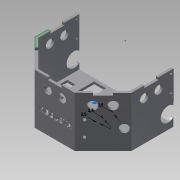
# Autodesk Inventor part: Kepala Depan 2
Saved by Autodesk Inventor 2015 SP1 (Build 190203100, 203)
## iProperties
Created: 2015-02-01
Part Number: Kepala Depan 2
Material: Generic
Document SubType Name: Modeling
Designer: Rafi Kurnia Putra
Density: 1 g/cm^3
Appearance: Default
Mass: 71.957 g
Surface Area: 473.113 cm^2
Volume: 71.957 cm^3
Author: Rafi Kurnia Putra
Autodesk Inventor part; units mm, degrees
ref_plane "YZ Plane" through (0, 0, 0) normal (1, 0, 0) x (0, 1, 0)
ref_plane "XZ Plane" through (0, 0, 0) normal (0, 1, 0) x (-1, 0, 0)
ref_plane "XY Plane" through (0, 0, 0) normal (0, 0, 1) x (1, 0, 0)
sketch "Sketch1" plane through (0, 0, 0) normal (0, 1, 0) x (-1, 0, 0)
  line L0 (60.406, -52.6639) -> (25.0211, -88.0488)
  line L1 (60.406, -52.6639) -> (60.406, 0)
  line L2 (-60.4057, -52.6639) -> (-60.4057, 0)
  line L3 (25.0211, -88.0488) -> (-25.0207, -88.0488)
  line L4 (-60.4057, 0) -> (60.406, 0)
  line L5 (-25.0207, -88.0488) -> (-60.4057, -52.6639)
  line L6 (57.406, 0) -> (57.406, -51.4212)
  line L7 (57.406, -51.4212) -> (23.7784, -85.0488)
  line L8 (23.7784, -85.0488) -> (-23.7781, -85.0488)
  line L9 (-23.7781, -85.0488) -> (-57.4057, -51.4212)
  line L10 (-57.4057, -51.4212) -> (-57.4057, 0)
  point P0 (0, -6165561.8884)
  point P1 (0, 0)
  point P2 (0.0002, 0)
  dimension "d195" = 120.8117
  dimension "d198" = 50.0418
  dimension "d199" = 50.0418
  dimension "d200" = 50.0418
  dimension "d201" = 52.6639
  dimension "d202" = 52.6639
  dimension "d204" = 3
  dimension "d205" = 51.4212
  dimension "d206" = 47.5566
  dimension "d207" = 47.5566
  dimension "d208" = 47.5566
  dimension "d209" = 51.4212
  dimension "d210" = 135
  dimension "d211" = 135
  dimension "d212" = 135
  dimension "d213" = 135
  dimension "d214" = 135
  dimension "d215" = 135
  dimension "d216" = 135
  dimension "d217" = 135
  dimension "d218" = 3
  dimension "d219" = 3
  dimension "d220" = 3
  constraints: 22 end point, 2 point on line, 1 horizontal, 1 horizontal alignment, 1 midpoint, 1 vertical, 3 other
  measures "d195" distance between parallel lines of L2 L1
  measures "d198" distance of L0.end L3.end
  measures "d199" distance of L0.start L0.end
  measures "d200" distance of L3.end L2.start
  measures "d201" distance of L0.start L1.end
  measures "d202" distance of L2.start L2.end
  measures "d204" distance between parallel lines of L6 L1
  measures "d205" distance of L6.start L6.end
  measures "d206" distance of L6.end L7.end
  measures "d207" distance of L7.end L8.end
  measures "d208" distance of L8.end L9.end
  measures "d209" distance of L9.end L10.end
  measures "d210" angle of L7 L6
  measures "d211" angle of L8 L7
  measures "d212" angle of L9 L8
  measures "d213" angle of L10 L9
  measures "d214" angle of L0 L1
  measures "d215" angle of L3 L0
  measures "d216" angle of L5 L3
  measures "d217" angle of L2 L5
  measures "d218" distance between parallel lines of L7 L0
  measures "d219" distance between parallel lines of L8 L3
  measures "d220" distance between parallel lines of L5 L9
extrude "Extrusion8" add sketch "Sketch1" along normal blind 3
extrude "Extrusion9" add sketch "Sketch1" against normal blind 60 contours L0 L3 L5 L2 L4 L10 L9 L8 L7 L6 L1
sketch "Sketch10" plane through (0, 3, 0) normal (0, 1, 0) x (1, 0, 0)
  circle A0 centre (13.2193, 32.61) radius 1.75
  circle A1 centre (39.7053, 32.61) radius 1.75
  circle A2 centre (39.7053, 8.2) radius 1.75
  circle A3 centre (13.2193, 8.2) radius 1.75
  circle A4 centre (20, 57.8773) radius 1.75
  circle A5 centre (-20, 57.8773) radius 1.75
  point P0 (0, 0)
  dimension "d115" = 3.5
  dimension "d116" = 3.5
  dimension "d117" = 3.5
  dimension "d118" = 3.5
  dimension "d119" = 3.5
  dimension "d120" = 3.5
  constraints: 6 centre point, 1 coincident
  measures "d115" diameter of A0
  measures "d116" diameter of A1
  measures "d117" diameter of A2
  measures "d118" diameter of A3
  measures "d119" diameter of A4
  measures "d120" diameter of A5
extrude "Extrusion10" cut sketch "Sketch10" against normal up to next
sketch "Sketch11" plane through (0, 3, 0) normal (0, 1, 0) x (1, 0, 0)
  line L0 (53.5557, 36.3929) -> (43.5557, 36.3929)
  line L1 (43.5557, 36.3929) -> (43.5557, 18.8929)
  line L2 (43.5557, 18.8929) -> (53.5557, 18.8929)
  line L3 (53.5557, 18.8929) -> (53.5557, 36.3929)
  line L4 (53.5557, 36.3929) -> (43.5557, 18.8929) construction
  line L5 (43.5557, 36.3929) -> (53.5557, 18.8929) construction
  line L6 (-53.5557, 36.3929) -> (-43.5557, 36.3929)
  line L7 (-43.5557, 36.3929) -> (-43.5557, 18.8929)
  line L8 (-43.5557, 18.8929) -> (-53.5557, 18.8929)
  line L9 (-53.5557, 18.8929) -> (-53.5557, 36.3929)
  line L10 (-53.5557, 36.3929) -> (-43.5557, 18.8929) construction
  line L11 (-43.5557, 36.3929) -> (-53.5557, 18.8929) construction
  line L12 (-8.75, 82.4488) -> (8.75, 82.4488)
  line L13 (8.75, 82.4488) -> (8.75, 67.4488)
  line L14 (8.75, 67.4488) -> (-8.75, 67.4488)
  line L15 (-8.75, 67.4488) -> (-8.75, 82.4488)
  line L16 (-8.75, 82.4488) -> (8.75, 67.4488) construction
  line L17 (8.75, 82.4488) -> (-8.75, 67.4488) construction
  line L18 (36.9856, 52.2544) -> (24.6113, 64.6288)
  line L19 (24.6113, 64.6288) -> (31.6823, 71.6998)
  line L20 (31.6823, 71.6998) -> (44.0567, 59.3254)
  line L21 (44.0567, 59.3254) -> (36.9856, 52.2544)
  line L22 (36.9856, 52.2544) -> (31.6823, 71.6998) construction
  line L23 (24.6113, 64.6288) -> (44.0567, 59.3254) construction
  line L24 (-44.057, 59.3254) -> (-31.6827, 71.6998)
  line L25 (-31.6827, 71.6998) -> (-24.6116, 64.6288)
  line L26 (-24.6116, 64.6288) -> (-36.986, 52.2544)
  line L27 (-36.986, 52.2544) -> (-44.057, 59.3254)
  line L28 (-44.057, 59.3254) -> (-24.6116, 64.6288) construction
  line L29 (-31.6827, 71.6998) -> (-36.986, 52.2544) construction
  line L30 (-23.7595, 81.9564) -> (-54.3136, 51.4023)
  line L31 (-23.7595, 81.9564) -> (-24.9616, 83.1585)
  line L32 (-54.3136, 51.4023) -> (-55.5157, 52.6044)
  line L33 (-24.9616, 83.1585) -> (-54.3136, 51.4023)
  line L34 (-55.5157, 52.6044) -> (-23.7595, 81.9564)
  line L35 (-39.6376, 67.2804) -> (60.3624, 67.2804) construction
  line L36 (-55.206, 49.2479) -> (-55.206, 6.0379)
  line L37 (21.6048, 82.8488) -> (-21.6052, 82.8488)
  line L38 (54.3133, 51.4023) -> (23.7592, 81.9564)
  line L39 (55.2057, 6.0379) -> (55.2057, 49.2479)
  point P0 (0, 0)
  point P1 (48.5557, 27.6429)
  point P2 (-48.5557, 27.6429)
  point P3 (0, 74.9488)
  point P4 (-2.6515, 135.1442)
  point P5 (34.334, 61.9771)
  point P6 (-34.3343, 61.9771)
  point P7 (-34.3343, 61.9771)
extrude "Extrusion11" cut sketch "Sketch11" against normal up to next contours L3 L2 L1 L0 | L6 L7 L8 L9 | L12 L13 L14 L15 | L18 L19 L20 L21 | L24 L25 L26 L27
sketch "Sketch12" plane through (0, 3, 0) normal (0, 1, 0) x (1, 0, 0)
  circle A0 centre (-37.593, 41.7496) radius 1.75 projected
  circle A1 centre (37.593, 41.7496) radius 1.75 projected
  point P0 (0, 0)
extrude "Extrusion12" cut sketch "Sketch12" against normal up to next
sketch "Sketch18" plane through (0, 0, 0) normal (0, -1, 0) x (1, 0, 0)
  circle A0 centre (49.9057, -48.3146) radius 1.75
  circle A1 centre (-49.906, -48.3146) radius 1.75
  line L0 (-56.906, -51.2141) -> (-56.906, 0) projected
  line L1 (-23.5713, -84.5488) -> (-56.906, -51.2141) projected
  line L2 (56.9057, 0) -> (56.9057, -51.2141) projected
  line L3 (56.9057, -51.2141) -> (23.571, -84.5488) projected
  point P0 (0, 0)
  dimension "d161" = 3.5
  dimension "d162" = 3.5
  dimension "d163" = 7
  dimension "d164" = 7
  dimension "d165" = 7
  dimension "d166" = 7
  constraints: 2 centre point
  measures "d161" diameter of A0
  measures "d162" diameter of A1
  measures "d163" distance from line of L1 A1.centre
  measures "d164" distance from line of A1.centre L0
  measures "d165" distance from line of A0.centre L2
  measures "d166" distance from line of L3 A0.centre
extrude "Extrusion19" cut sketch "Sketch18" against normal up to next
sketch "Sketch20" plane through (60.4057, 3, 0) normal (1, 0, 0) x (0, 0, -1)
  circle A0 centre (3, -59.0338) radius 1 projected
  circle A1 centre (3, -38.0338) radius 1 projected
  point P0 (0, -3)
extrude "Extrusion22" cut sketch "Sketch20" against normal through all
sketch "Sketch21" plane through (0, 3, 0) normal (0, 1, 0) x (1, 0, 0)
  line L0 (-25.1532, 6.0483) -> (-25.1532, 26.3545)
  line L1 (-30.1532, 7.5789) -> (-30.1532, 26.3545)
  line L2 (-25.1532, 26.3545) -> (-30.1532, 26.3545)
  line L3 (-25.1532, 6.0483) -> (-30.1532, 6.0483)
  line L4 (-30.1532, 6.0483) -> (-30.1532, 7.5789)
  line L5 (-22.6532, 3.8312) -> (-32.6532, 3.8312)
  line L6 (-32.6532, 3.8312) -> (-32.6532, 28.5716)
  line L7 (-32.6532, 28.5716) -> (-22.6532, 28.5716)
  line L8 (-22.6532, 28.5716) -> (-22.6532, 3.8312)
  line L9 (-22.6532, 3.8312) -> (-32.6532, 28.5716) construction
  line L10 (-32.6532, 3.8312) -> (-22.6532, 28.5716) construction
  point P0 (0, 0)
  point P1 (-27.6532, 16.2014)
  dimension "d329" = 10
  constraints: 22 end point, 3 horizontal, 2 midpoint, 2 parallel, 2 perpendicular
  measures "d329" distance of L6.end L7.end
extrude "Extrusion23" cut sketch "Sketch21" against normal up to next contours L3 L4 L1 L2 L0 | L5 L6 L7 L8
sketch "Sketch22" plane through (0, -60, 0) normal (0, -1, 0) x (1, 0, 0)
  line L0 (57.406, -36.3929) -> (60.406, -36.3929)
  line L1 (57.406, -18.8928) -> (60.406, -18.8929)
  line L2 (57.406, -18.8928) -> (60.406, -18.8928) construction
  line L3 (60.406, -18.8929) -> (60.406, -36.3929)
  line L4 (57.406, -36.3929) -> (57.406, -18.8928)
  line L5 (34.4047, -74.4222) -> (36.526, -76.5435)
  line L6 (46.7791, -62.0478) -> (48.9004, -64.1691)
  line L7 (36.526, -76.5435) -> (48.9004, -64.1691)
  line L8 (46.7791, -62.0478) -> (34.4047, -74.4222)
  line L9 (-8.7498, -88.0488) -> (-8.7498, -85.0488)
  line L10 (0, 0) -> (0, -8)
  line L11 (-57.406, -36.3929) -> (-60.406, -36.3929)
  line L12 (-57.406, -18.8928) -> (-60.406, -18.8929)
  line L13 (-57.406, -18.8928) -> (-60.406, -18.8928) construction
  line L14 (-60.406, -18.8929) -> (-60.406, -36.3929)
  line L15 (-57.406, -36.3929) -> (-57.406, -18.8928)
  line L16 (-34.4047, -74.4222) -> (-36.526, -76.5435)
  line L17 (-46.7791, -62.0478) -> (-48.9004, -64.1691)
  line L18 (-36.526, -76.5435) -> (-48.9004, -64.1691)
  line L19 (-46.7791, -62.0478) -> (-34.4047, -74.4222)
  line L20 (8.7498, -88.0488) -> (8.7498, -85.0488)
  line L21 (-57.406, 0) -> (-60.406, 0) projected
  line L22 (-60.406, 0) -> (-60.406, -52.6639) projected
  line L23 (-60.406, -52.6639) -> (-25.0211, -88.0488) projected
  line L24 (-25.0211, -88.0488) -> (25.0207, -88.0488) projected
  line L25 (25.0207, -88.0488) -> (60.4057, -52.6639) projected
  line L26 (60.4057, -52.6639) -> (60.4057, 0) projected
  line L27 (60.4057, 0) -> (57.4057, 0) projected
  line L28 (57.4057, 0) -> (57.4057, -51.4212) projected
  line L29 (57.4057, -51.4212) -> (23.7781, -85.0488) projected
  line L30 (23.7781, -85.0488) -> (-23.7784, -85.0488) projected
  line L31 (-23.7784, -85.0488) -> (-57.406, -51.4212) projected
  line L32 (-57.406, -51.4212) -> (-57.406, 0) projected
  line L33 (-60.406, 0) -> (-60.406, -52.6639) projected
  line L34 (60.4057, -52.6639) -> (60.4057, 0) projected
  line L35 (23.7781, -85.0488) -> (-23.7784, -85.0488) projected
  line L36 (8.7498, -88.0488) -> (-8.7498, -88.0488)
  line L37 (8.7498, -85.0488) -> (-8.7498, -85.0488)
  line L38 (36.9856, -52.2544) -> (44.0567, -59.3254) projected
  line L39 (31.6823, -71.6998) -> (24.6113, -64.6288) projected
  line L40 (53.5557, -36.3929) -> (43.5557, -36.3929) projected
  line L41 (-43.5557, -36.3929) -> (-53.5557, -36.3929) projected
  point P0 (-0.0002, -87)
  dimension "d181" = 17.5
  dimension "d221" = 3
  dimension "d222" = 0
  dimension "d223" = 17.5001
  dimension "d225" = 3
  dimension "d231" = 0
  constraints: 46 end point, 11 symmetric about line, 5 collinear, 3 horizontal, 2 parallel, 1 equal length, 1 horizontal alignment, 1 perpendicular, 1 other
  measures "d181" distance of L12.end L11.end
  measures "d221" distance between parallel lines of L14 L15
  measures "d222" distance from line of L22 L11.end
  measures "d223" distance of L1.start L0.start
  measures "d225" distance of L16.start L16.end
  measures "d231" distance between parallel lines of L36 L24
sketch "Sketch23" plane through (0, 3, 0) normal (0, 1, 0) x (1, 0, 0)
  circle A0 centre (-27.94, 46.62) radius 1.75 projected
  circle A1 centre (43, 59.9982) radius 1.75 projected
  circle A2 centre (-27.94, 46.62) radius 1.5875 projected
  circle A3 centre (20.32, 40.27) radius 1.5875 projected
  point P0 (0, 0)
extrude "Extrusion27" cut sketch "Sketch23" against normal up to next contours A2 | A3
sketch "Sketch26" plane through (25.0207, 3, -88.0488) normal (0, 0, -1) x (-1, 0, 0)
  line L0 (14.0407, -9.138) -> (36.0007, -9.138) projected
  line L1 (36.0007, -4.158) -> (14.0407, -4.158) projected
  line L2 (36.5007, -8.638) -> (36.5007, -4.658) projected
  line L3 (13.5407, -4.658) -> (13.5407, -8.638) projected
  arc A0 (13.5407, -8.638) -> (14.0407, -9.138) centre (14.0407, -8.638) ccw projected
  arc A1 (36.0007, -9.138) -> (36.5007, -8.638) centre (36.0007, -8.638) ccw projected
  arc A2 (36.5007, -4.658) -> (36.0007, -4.158) centre (36.0007, -4.658) ccw projected
  arc A3 (14.0407, -4.158) -> (13.5407, -4.658) centre (14.0407, -4.658) ccw projected
  line L4 (14.0407, -2) -> (36.0007, -2)
  arc A4 (38.6587, -4.658) -> (36.0007, -2) centre (36.0007, -4.658) ccw
  line L5 (38.6587, -4.658) -> (38.6587, -8.638)
  arc A5 (36.0007, -11.296) -> (38.6587, -8.638) centre (36.0007, -8.638) ccw
  line L6 (36.0007, -11.296) -> (14.0407, -11.296)
  arc A6 (11.3827, -8.638) -> (14.0407, -11.296) centre (14.0407, -8.638) ccw
  line L7 (11.3827, -8.638) -> (11.3827, -4.658)
  arc A7 (14.0407, -2) -> (11.3827, -4.658) centre (14.0407, -4.658) ccw
  point P0 (25.0207, -3)
  constraints: 8 end point, 8 point on circle, 4 centre point, 7 other
extrude "Extrusion30" [suppressed]
extrude "Extrusion31" cut sketch "Sketch22" against normal blind 3 contours L4 L1 L3 L0 | L6 L7 L5 L8 | L20 L24 L9 L30 | L16 L18 L17 L19 | L11 L14 L12 L15
sketch "Sketch27" plane through (-60.406, -60, -52.6639) normal (-0.7071068, 0, -0.7071068) x (-0.7071068, 0, 0.7071068)
  line L0 (-33.7712, 3) -> (-16.2712, 3) projected
  line L1 (-16.2712, 0) -> (-16.2712, 3) projected
  line L2 (-33.7712, 0) -> (-33.7712, 3) projected
  line L3 (0, 0) -> (-50.0418, 0) projected
  point P0 (-5.4745, 60)
extrude "Extrusion32" cut sketch "Sketch27" against normal blind 3
sketch "Sketch28" plane through (57.406, -60, -18.8928) normal (1, 0, 0) x (0, 0, -1)
  line L0 (17.5001, 0) -> (0, 0) projected
  line L1 (17.5001, 0) -> (17.5001, 3) projected
  line L2 (17.5001, 3) -> (0, 3) projected
  line L3 (0, 0) -> (0, 3) projected
  point P0 (-18.8928, 60)
extrude "Extrusion33" cut sketch "Sketch28" along normal mid plane 3
sketch "Sketch31" plane through (0, 3, 0) normal (0, 1, 0) x (1, 0, 0)
  circle A0 centre (20.32, 40.27) radius 1.5875 projected
  circle A1 centre (20.32, 40.27) radius 1.75
  circle A2 centre (37.593, 41.7496) radius 1.75 projected
  circle A3 centre (-27.94, 46.62) radius 1.5875 projected
  circle A4 centre (-27.94, 46.62) radius 1.5875 projected
  circle A5 centre (-27.94, 46.62) radius 1.75
  point P0 (0, 0)
  dimension "d242" = 3.5
  dimension "d243" = 3.5
  constraints: 2 centre point, 2 coincident
  measures "d242" diameter of A1
  measures "d243" diameter of A5
extrude "Extrusion36" cut sketch "Sketch31" against normal up to next contours A1 | A5
sketch "Sketch34" plane through (25.0207, 3, -88.0488) normal (0, 0, -1) x (-1, 0, 0)
  circle A0 centre (16.0209, -49.2838) radius 5.125
  circle A1 centre (34.0209, -49.2838) radius 5.125
  point P0 (25.0207, -3)
  point P1 (25.0209, -49.2838)
  dimension "d270" = 10.25
  dimension "d271" = 10.25
  dimension "d272" = 18
  dimension "d273" = 9
  constraints: 2 centre point, 1 other
  measures "d270" diameter of A0
  measures "d271" diameter of A1
  measures "d272" distance of A0.centre A1.centre
  measures "d273" distance of point (25.021, -49.284) A1.centre
sketch "Sketch35" plane through (25.0207, -60, -88.0488) normal (0.7071068, 0, -0.7071068) x (-0.7071068, 0, -0.7071068)
  circle A0 centre (-34.0209, 13.7162) radius 5.125
  circle A1 centre (-16.0209, 13.7162) radius 5.125
  point P0 (-44.5675, 60)
  point P1 (-25.0209, 13.7162)
  dimension "d276" = 10.25
  dimension "d277" = 10.25
  dimension "d278" = 9
  dimension "d279" = 9
  constraints: 2 centre point, 1 other
  measures "d276" diameter of A0
  measures "d277" diameter of A1
  measures "d278" distance of point (-25.021, 13.716) A1.centre
  measures "d279" distance of point (-25.021, 13.716) A0.centre
sketch "Sketch36" plane through (60.4057, 3, 0) normal (1, 0, 0) x (0, 0, -1)
  circle A0 centre (18.6429, -49.2838) radius 5.125
  circle A1 centre (36.6429, -49.2838) radius 5.125
  point P0 (0, -3)
  point P1 (27.6429, -49.2838)
  dimension "d282" = 10.25
  dimension "d283" = 10.25
  dimension "d284" = 18
  dimension "d285" = 9
  constraints: 2 centre point, 1 other
  measures "d282" diameter of A0
  measures "d283" diameter of A1
  measures "d284" distance of A0.centre A1.centre
  measures "d285" distance of point (27.643, -49.284) A1.centre
sketch "Sketch37" plane through (-60.406, -60, -52.6639) normal (-0.7071068, 0, -0.7071068) x (-0.7071068, 0, 0.7071068)
  circle A0 centre (-34.0209, 13.7162) radius 5.125
  circle A1 centre (-16.0209, 13.7162) radius 5.125
  point P0 (-5.4745, 60)
  point P1 (-25.0209, 13.7162)
  dimension "d289" = 10.25
  dimension "d290" = 10.25
  dimension "d291" = 18
  dimension "d292" = 9
  constraints: 2 centre point, 1 other
  measures "d289" diameter of A0
  measures "d290" diameter of A1
  measures "d291" distance of A0.centre A1.centre
  measures "d292" distance of point (-25.021, 13.716) A1.centre
sketch "Sketch38" plane through (60.4057, 3, 0) normal (1, 0, 0) x (0, 0, -1)
  circle A0 centre (6.7939, -16.9) radius 9.2 projected
  point P0 (0, -3)
extrude "Extrusion44" cut sketch "Sketch38" against normal through all
sketch "Sketch40" plane through (0, 0, 0) normal (0, -1, 0) x (1, 0, 0)
  circle A0 centre (12, -46) radius 1.75
  circle A1 centre (12, -26.5036) radius 1.75
  line L0 (0, -56) -> (0, -18) construction
  circle A2 centre (-12, -46) radius 1.75
  circle A3 centre (-12, -26.5036) radius 1.75
  circle A4 centre (12, -38.5036) radius 1.75
  circle A5 centre (-12, -38.5036) radius 1.75
  point P0 (0, 0)
  dimension "d262" = 3.5
  dimension "d263" = 3.5
  dimension "d340" = 3.5
  constraints: 6 centre point, 2 end point, 1 symmetric about line, 1 vertical, 1 other
  measures "d262" diameter of A0
  measures "d263" diameter of A1
  measures "d340" diameter of A4
sketch "Sketch46" plane through (0, 0, 0) normal (0, -1, 0) x (1, 0, 0)
  line L0 (-32.6532, -28.5716) -> (-32.6532, -3.8312) projected
  line L1 (-32.6532, -3.8312) -> (-22.6532, -3.8312) projected
  line L2 (-32.6532, -3.8312) -> (-37.6532, -3.8312)
  line L3 (-37.6532, -3.8312) -> (-37.6532, -28.5716)
  line L4 (-37.6532, -28.5716) -> (-32.6532, -28.5716)
  line L5 (-32.6532, -28.5716) -> (-32.6532, -3.8312)
  line L6 (8.75, -67.4488) -> (-8.75, -67.4488)
  line L7 (-8.75, -67.4488) -> (-8.75, -57.4488)
  line L8 (-8.75, -57.4488) -> (8.75, -57.4488)
  line L9 (8.75, -57.4488) -> (8.75, -67.4488)
  point P0 (0, 0)
  dimension "d330" = 5
  dimension "d331" = 10
  constraints: 16 end point, 4 parallel, 2 horizontal, 2 perpendicular
  measures "d330" distance of L4.end L3.end
  measures "d331" distance of L6.end L7.end
sketch "Sketch41" plane through (0, -60, 0) normal (0, -1, 0) x (1, 0, 0)
  line L0 (-48.9006, -64.1693) -> (-46.7792, -62.048) projected
  line L1 (-46.7792, -62.048) -> (-57.406, -51.4212) projected
  line L2 (-57.406, -51.4212) -> (-57.406, -36.3929) projected
  line L3 (-57.406, -36.3929) -> (-60.406, -36.3929) projected
  line L4 (-60.406, -36.3929) -> (-60.406, -52.6639) projected
  line L5 (-60.406, -52.6639) -> (-48.9006, -64.1693) projected
  point P0 (0, 0)
sketch "Sketch42" plane through (25.0207, -60, -88.0488) normal (0.7071068, 0, -0.7071068) x (-0.7071068, 0, -0.7071068)
  line L0 (-16.2709, 3) -> (-16.2709, 0) projected
  line L1 (0, 0) -> (-16.2709, 0) projected
  line L2 (0, 0) -> (0, 63) projected
  line L3 (-50.0418, 63) -> (0, 63) projected
  line L4 (-50.0418, 0) -> (-50.0418, 63) projected
  line L5 (-33.7709, 0) -> (-50.0418, 0) projected
  line L6 (-33.7709, 0) -> (-33.7709, 3) projected
  line L7 (-33.7709, 3) -> (-16.2709, 3) projected
  circle A0 centre (-8.542, 29.25) radius 1.75
  circle A1 centre (-8.542, 48) radius 1.75
  line L8 (-48.7992, 60) -> (-48.7992, 0) projected
  circle A2 centre (-43.7992, 38.625) radius 5
  point P0 (-44.5675, 60)
  dimension "d293" = 3.5
  dimension "d294" = 3.5
  dimension "d295" = 18.75
  dimension "d296" = 29.25
  dimension "d297" = 8.542
  dimension "d307" = 10
  dimension "d308" = 5
  dimension "d309" = 9.375
  constraints: 3 centre point
  measures "d293" diameter of A0
  measures "d294" diameter of A1
  measures "d295" distance of A1.centre A0.centre
  measures "d296" distance from line of A0.centre L1
  measures "d297" distance from line of A0.centre L2
  measures "d307" diameter of A2
  measures "d308" distance from line of A2.centre L8
  measures "d309" vertical distance of A2.centre A0.centre
sketch "Sketch43" plane through (-60.406, -60, -52.6639) normal (-0.7071068, 0, -0.7071068) x (-0.7071068, 0, 0.7071068)
  line L0 (-33.7712, 0) -> (-33.7712, 3) projected
  line L1 (-33.7712, 3) -> (-16.2712, 3) projected
  line L2 (-16.2712, 3) -> (-16.2712, 0) projected
  line L3 (0, 0) -> (-16.2712, 0) projected
  line L4 (0, 0) -> (0, 63) projected
  line L5 (-50.0418, 63) -> (0, 63) projected
  line L6 (-50.0418, 0) -> (-50.0418, 63) projected
  line L7 (-33.7712, 0) -> (-50.0418, 0) projected
  circle A0 centre (-41.4998, 29.25) radius 1.75
  circle A1 centre (-41.4998, 48) radius 1.75
  circle A2 centre (-6.2426, 38.625) radius 5
  line L8 (-1.2426, 60) -> (-1.2426, 0) projected
  point P0 (-5.4745, 60)
  dimension "d298" = 3.5
  dimension "d299" = 3.5
  dimension "d300" = 8.542
  dimension "d301" = 8.542
  dimension "d302" = 18.75
  dimension "d303" = 29.25
  dimension "d304" = 10
  dimension "d305" = 9.375
  dimension "d306" = 5
  constraints: 3 centre point
  measures "d298" diameter of A0
  measures "d299" diameter of A1
  measures "d300" distance from line of L6 A0.centre
  measures "d301" distance from line of L6 A1.centre
  measures "d302" distance of A1.centre A0.centre
  measures "d303" distance from line of L7 A0.centre
  measures "d304" diameter of A2
  measures "d305" vertical distance of A2.centre A0.centre
  measures "d306" distance from line of A2.centre L8
sketch "Sketch44" plane through (0, 0, 0) normal (0, -1, 0) x (1, 0, 0)
  circle A0 centre (21, -46) radius 1.75 projected
  circle A1 centre (20, -57.8773) radius 1.75 projected
  circle A2 centre (-21, -46) radius 1.75 projected
  circle A3 centre (-20, -57.8773) radius 1.75 projected
  circle A4 centre (20, -51.8773) radius 1.75
  circle A5 centre (-20, -51.8773) radius 1.75
  point P0 (0, 0)
  dimension "d310" = 11.8773
  dimension "d311" = 6
  dimension "d312" = 6
  constraints: 2 centre point
  measures "d310" vertical distance of A0.centre A1.centre
  measures "d311" distance of A4.centre A1.centre
  measures "d312" distance of A5.centre A3.centre
extrude "Extrusion46" cut sketch "Sketch36" against normal through all
extrude "Extrusion47" cut sketch "Sketch35" against normal through all
extrude "Extrusion48" cut sketch "Sketch42" against normal through all contours A0 | A1 | A2
extrude "Extrusion49" cut sketch "Sketch34" against normal through all
extrude "Extrusion50" cut sketch "Sketch37" against normal up to next
extrude "Extrusion51" cut sketch "Sketch43" against normal up to next contours A0 | A1 | A2
extrude "Extrusion52" cut sketch "Sketch44" against normal through all contours A4 | A5
extrude "Extrusion54" cut sketch "Sketch46" against normal through all contours L6 L7 L8 L9
extrude "Extrusion55" cut sketch "Sketch40" against normal blind 10 contours A0 | A1 | A2 | A3
sketch "Sketch47" plane through (25.0207, 3, -88.0488) normal (0, 0, -1) x (-1, 0, 0)
  line L0 (45.0523, -27.4707) -> (24.2423, -27.4707) construction
  line L1 (24.2423, -27.4707) -> (24.2423, -23.8233) construction
  line L2 (24.2423, -23.8233) -> (45.0523, -23.8233) construction
  line L3 (45.0523, -23.8233) -> (45.0523, -27.4707) construction
  circle A0 centre (16.0209, -49.2838) radius 5.125 projected
  circle A1 centre (34.0209, -49.2838) radius 5.125 projected
  line L4 (33.7706, -60) -> (33.7706, -63) projected
  line L5 (50.0418, -63) -> (33.7706, -63) projected
  line L6 (50.0418, -63) -> (50.0418, 0) projected
  line L7 (0, 0) -> (50.0418, 0) projected
  line L8 (0, -63) -> (0, 0) projected
  line L9 (16.2709, -63) -> (0, -63) projected
  line L10 (16.2709, -63) -> (16.2709, -60) projected
  line L11 (16.2709, -60) -> (33.7706, -60) projected
  line L12 (38.7842, -21.2422) -> (40.6479, -21.2422)
  line L13 (40.6479, -21.2422) -> (42.3434, -23.4815)
  line L14 (42.3434, -23.4815) -> (42.897, -23.4815)
  line L15 (42.897, -23.4815) -> (42.897, -21.2422)
  line L16 (42.897, -21.2422) -> (44.4196, -21.2422)
  line L17 (44.4196, -21.2422) -> (44.4196, -27.3422)
  line L18 (44.4196, -27.3422) -> (41.9677, -27.3422)
  spline S0 degree 2 poles (41.9677, -27.3422) (41.4586, -27.3422) (40.7072, -27.2137) (40.3859, -27.016) knots 0 0 0 1 2 2 2
  spline S1 degree 2 poles (40.3859, -27.016) (40.0596, -26.8083) (39.674, -26.1608) (39.674, -25.6664) knots 0 0 0 1 2 2 2
  spline S2 degree 2 poles (39.674, -25.6664) (39.674, -24.9694) (40.3068, -24.0945) (40.8357, -23.8374) knots 0 0 0 1 2 2 2
  line L19 (40.8357, -23.8374) -> (38.7842, -21.2422)
  spline S3 degree 2 poles (41.246, -25.4737) (41.246, -25.706) (41.4239, -26.0372) (41.6266, -26.1262) knots 0 0 0 1 2 2 2
  spline S4 degree 2 poles (41.6266, -26.1262) (41.77, -26.1855) (42.121, -26.2201) (42.3829, -26.2201) knots 0 0 0 1 2 2 2
  line L20 (42.3829, -26.2201) -> (42.897, -26.2201)
  line L21 (42.897, -26.2201) -> (42.897, -24.5789)
  line L22 (42.897, -24.5789) -> (42.4571, -24.5789)
  spline S5 degree 2 poles (42.4571, -24.5789) (42.1407, -24.5789) (41.6909, -24.658) (41.5376, -24.7816) knots 0 0 0 1 2 2 2
  spline S6 degree 2 poles (41.5376, -24.7816) (41.3893, -24.9002) (41.246, -25.2166) (41.246, -25.4737) knots 0 0 0 1 2 2 2
  spline S7 degree 2 poles (32.7782, -24.2922) (32.7782, -22.8092) (34.36, -21.1137) (35.7342, -21.1137) knots 0 0 0 1 2 2 2
  spline S8 degree 2 poles (35.7342, -21.1137) (37.1134, -21.1137) (38.6854, -22.829) (38.6854, -24.2922) knots 0 0 0 1 2 2 2
  spline S9 degree 2 poles (38.6854, -24.2922) (38.6854, -25.7604) (37.1134, -27.4707) (35.7342, -27.4707) knots 0 0 0 1 2 2 2
  spline S10 degree 2 poles (35.7342, -27.4707) (34.36, -27.4707) (32.7782, -25.7703) (32.7782, -24.2922) knots 0 0 0 1 2 2 2
  spline S11 degree 2 poles (34.36, -24.2922) (34.36, -24.8409) (34.5825, -25.6071) (34.7752, -25.8493) knots 0 0 0 1 2 2 2
  spline S12 degree 2 poles (34.7752, -25.8493) (34.968, -26.1015) (35.4624, -26.319) (35.7293, -26.319) knots 0 0 0 1 2 2 2
  spline S13 degree 2 poles (35.7293, -26.319) (36.0111, -26.319) (36.4708, -26.1163) (36.6833, -25.8592) knots 0 0 0 1 2 2 2
  spline S14 degree 2 poles (36.6833, -25.8592) (36.8712, -25.622) (37.1035, -24.836) (37.1035, -24.2922) knots 0 0 0 1 2 2 2
  spline S15 degree 2 poles (37.1035, -24.2922) (37.1035, -23.7287) (36.8811, -22.9872) (36.6883, -22.7351) knots 0 0 0 1 2 2 2
  spline S16 degree 2 poles (36.6883, -22.7351) (36.4955, -22.483) (35.9962, -22.2655) (35.7293, -22.2655) knots 0 0 0 1 2 2 2
  spline S17 degree 2 poles (35.7293, -22.2655) (35.4574, -22.2655) (34.9532, -22.4978) (34.7703, -22.745) knots 0 0 0 1 2 2 2
  spline S18 degree 2 poles (34.7703, -22.745) (34.5726, -23.0119) (34.36, -23.7188) (34.36, -24.2922) knots 0 0 0 1 2 2 2
  spline S19 degree 2 poles (26.9945, -23.1108) (26.9945, -22.656) (27.3406, -21.9689) (27.6273, -21.7415) knots 0 0 0 1 2 2 2
  spline S20 degree 2 poles (27.6273, -21.7415) (27.9733, -21.4696) (28.7939, -21.2422) (29.4316, -21.2422) knots 0 0 0 1 2 2 2
  line L23 (29.4316, -21.2422) -> (31.8686, -21.2422)
  line L24 (31.8686, -21.2422) -> (31.8686, -27.3422)
  line L25 (31.8686, -27.3422) -> (29.7183, -27.3422)
  spline S21 degree 2 poles (29.7183, -27.3422) (29.046, -27.3422) (28.3539, -27.2384) (28.0524, -27.0753) knots 0 0 0 1 2 2 2
  spline S22 degree 2 poles (28.0524, -27.0753) (27.7212, -26.9023) (27.3999, -26.3091) (27.3999, -25.9235) knots 0 0 0 1 2 2 2
  spline S23 degree 2 poles (27.3999, -25.9235) (27.3999, -25.4786) (27.8448, -24.7816) (28.2402, -24.6185) knots 0 0 0 1 2 2 2
  line L26 (28.2402, -24.6185) -> (28.2402, -24.5888)
  spline S24 degree 2 poles (28.2402, -24.5888) (27.6718, -24.4702) (26.9945, -23.7336) (26.9945, -23.1108) knots 0 0 0 1 2 2 2
  spline S25 degree 2 poles (28.5764, -23.1355) (28.5764, -23.4222) (28.8038, -23.7435) (29.0312, -23.8275) knots 0 0 0 1 2 2 2
  spline S26 degree 2 poles (29.0312, -23.8275) (29.1696, -23.8819) (29.659, -23.8918) (30.0643, -23.8918) knots 0 0 0 1 2 2 2
  line L27 (30.0643, -23.8918) -> (30.3461, -23.8918)
  line L28 (30.3461, -23.8918) -> (30.3461, -22.3545)
  line L29 (30.3461, -22.3545) -> (30.262, -22.3545)
  spline S27 degree 2 poles (30.262, -22.3545) (29.6688, -22.3545) (29.2141, -22.3693) (28.9768, -22.4731) knots 0 0 0 1 2 2 2
  spline S28 degree 2 poles (28.9768, -22.4731) (28.7692, -22.567) (28.5764, -22.913) (28.5764, -23.1355) knots 0 0 0 1 2 2 2
  spline S29 degree 2 poles (28.957, -25.622) (28.957, -25.7703) (29.1103, -26.0817) (29.2684, -26.1509) knots 0 0 0 1 2 2 2
  spline S30 degree 2 poles (29.2684, -26.1509) (29.4167, -26.2201) (29.832, -26.23) (30.2423, -26.23) knots 0 0 0 1 2 2 2
  line L30 (30.2423, -26.23) -> (30.3461, -26.23)
  line L31 (30.3461, -26.23) -> (30.3461, -24.9348)
  line L32 (30.3461, -24.9348) -> (30.1533, -24.9348)
  spline S31 degree 2 poles (30.1533, -24.9348) (29.7628, -24.9348) (29.4464, -24.9497) (29.2783, -25.0288) knots 0 0 0 1 2 2 2
  spline S32 degree 2 poles (29.2783, -25.0288) (29.0954, -25.1177) (28.957, -25.4193) (28.957, -25.622) knots 0 0 0 1 2 2 2
  spline S33 degree 2 poles (23.6479, -21.1137) (24.8788, -21.1137) (26.2036, -22.3001) (26.2036, -23.4469) knots 0 0 0 1 2 2 2
  line L33 (26.2036, -23.4469) -> (26.2036, -27.3422)
  line L34 (26.2036, -27.3422) -> (24.6712, -27.3422)
  line L35 (24.6712, -27.3422) -> (24.6712, -23.5359)
  spline S34 degree 2 poles (24.6712, -23.5359) (24.6712, -22.8982) (24.1917, -22.2754) (23.6479, -22.2754) knots 0 0 0 1 2 2 2
  spline S35 degree 2 poles (23.6479, -22.2754) (23.119, -22.2754) (22.6247, -22.8735) (22.6247, -23.5359) knots 0 0 0 1 2 2 2
  line L36 (22.6247, -23.5359) -> (22.6247, -27.3422)
  line L37 (22.6247, -27.3422) -> (21.0923, -27.3422)
  line L38 (21.0923, -27.3422) -> (21.0923, -23.4519)
  spline S36 degree 2 poles (21.0923, -23.4519) (21.0923, -22.3248) (22.3825, -21.1137) (23.6479, -21.1137) knots 0 0 0 1 2 2 2
  spline S37 degree 2 poles (18.0324, -21.1335) (18.7343, -21.1335) (19.7922, -21.4053) (20.247, -21.6031) knots 0 0 0 1 2 2 2
  line L39 (20.247, -21.6031) -> (20.247, -23.0564)
  line L40 (20.247, -23.0564) -> (20.1086, -23.0564)
  spline S38 degree 2 poles (20.1086, -23.0564) (19.6488, -22.6659) (18.5465, -22.2457) (18.0274, -22.2457) knots 0 0 0 1 2 2 2
  spline S39 degree 2 poles (18.0274, -22.2457) (17.894, -22.2457) (17.4639, -22.305) (17.3354, -22.3643) knots 0 0 0 1 2 2 2
  spline S40 degree 2 poles (17.3354, -22.3643) (17.1772, -22.4335) (16.9547, -22.6857) (16.9547, -22.8883) knots 0 0 0 1 2 2 2
  spline S41 degree 2 poles (16.9547, -22.8883) (16.9547, -23.1207) (17.3156, -23.4074) (17.5628, -23.4716) knots 0 0 0 1 2 2 2
  spline S42 degree 2 poles (17.5628, -23.4716) (17.8742, -23.5557) (18.5811, -23.699) (18.8925, -23.8078) knots 0 0 0 1 2 2 2
  spline S43 degree 2 poles (18.8925, -23.8078) (19.5994, -24.0549) (20.2124, -24.9002) (20.2124, -25.533) knots 0 0 0 1 2 2 2
  spline S44 degree 2 poles (20.2124, -25.533) (20.2124, -26.3882) (18.764, -27.451) (17.6765, -27.451) knots 0 0 0 1 2 2 2
  spline S45 degree 2 poles (17.6765, -27.451) (17.1327, -27.451) (16.0551, -27.2285) (15.6299, -27.0407) knots 0 0 0 1 2 2 2
  line L41 (15.6299, -27.0407) -> (15.6299, -25.6467)
  line L42 (15.6299, -25.6467) -> (15.7634, -25.6467)
  spline S46 degree 2 poles (15.7634, -25.6467) (16.1045, -25.9383) (17.0833, -26.3387) (17.5974, -26.3387) knots 0 0 0 1 2 2 2
  spline S47 degree 2 poles (17.5974, -26.3387) (17.8, -26.3387) (18.1164, -26.2794) (18.2944, -26.2003) knots 0 0 0 1 2 2 2
  spline S48 degree 2 poles (18.2944, -26.2003) (18.4377, -26.1361) (18.6453, -25.879) (18.6453, -25.7208) knots 0 0 0 1 2 2 2
  spline S49 degree 2 poles (18.6453, -25.7208) (18.6453, -25.4835) (18.3141, -25.2117) (17.8396, -25.1029) knots 0 0 0 1 2 2 2
  spline S50 degree 2 poles (17.8396, -25.1029) (17.5331, -25.0337) (16.9646, -24.9002) (16.6384, -24.7865) knots 0 0 0 1 2 2 2
  spline S51 degree 2 poles (16.6384, -24.7865) (16.0056, -24.5542) (15.3877, -23.7831) (15.3877, -23.1503) knots 0 0 0 1 2 2 2
  spline S52 degree 2 poles (15.3877, -23.1503) (15.3877, -22.2408) (16.8163, -21.1335) (18.0324, -21.1335) knots 0 0 0 1 2 2 2
  line L43 (13.4302, -21.2422) -> (13.4302, -26.1805)
  line L44 (13.4302, -26.1805) -> (15.2345, -26.1805)
  line L45 (15.2345, -26.1805) -> (15.2345, -27.3422)
  line L46 (15.2345, -27.3422) -> (10.0935, -27.3422)
  line L47 (10.0935, -27.3422) -> (10.0935, -26.1805)
  line L48 (10.0935, -26.1805) -> (11.8978, -26.1805)
  line L49 (11.8978, -26.1805) -> (11.8978, -21.2422)
  line L50 (11.8978, -21.2422) -> (13.4302, -21.2422)
  line L51 (10.1231, -21.2422) -> (8.0618, -27.3422)
  line L52 (8.0618, -27.3422) -> (6.391, -27.3422)
  line L53 (6.391, -27.3422) -> (4.3296, -21.2422)
  line L54 (4.3296, -21.2422) -> (5.9065, -21.2422)
  line L55 (5.9065, -21.2422) -> (6.2872, -22.4879)
  line L56 (6.2872, -22.4879) -> (8.2051, -22.4879)
  line L57 (8.2051, -22.4879) -> (8.5907, -21.2422)
  line L58 (8.5907, -21.2422) -> (10.1231, -21.2422)
  line L59 (6.6233, -23.5952) -> (7.2462, -25.6121)
  line L60 (7.2462, -25.6121) -> (7.8739, -23.5952)
  line L61 (7.8739, -23.5952) -> (6.6233, -23.5952)
  point P0 (25.0207, -3)
  constraints: 2 other
extrude "Extrusion56" cut sketch "Sketch47" against normal blind 10 contours L12 L13 L14 L15 L16 L17 L18 S0 S1 S2 L19 | S7 S8 S9 S10 | S19 S20 L23 L24 L25 S21 S22 S23 L26 S24 | S33 L33 L34 L35 S34 S35 L36 L37 L38 S36 | S37 L39 L40 S38 S39 S40 S41 S42 S43 S44 S45 L41 L42 S46 S47 S48 S49 S50 S51 S52 | L43 L44 L45 L46 L47 L48 L49 L50 | L51 L52 L53 L54 L55 L56 L57 L58
sketch "Sketch48" plane through (25.0207, 3, -88.0488) normal (0, 0, -1) x (-1, 0, 0)
  spline S0 degree 2 poles (41.6266, -26.1262) (41.77, -26.1855) (42.121, -26.2201) (42.3829, -26.2201) knots 0 0 0 0.5 1 1 1 projected
  line L0 (42.3829, -26.2201) -> (42.897, -26.2201) projected
  line L1 (42.897, -26.2201) -> (42.897, -24.5789) projected
  line L2 (42.897, -24.5789) -> (42.4571, -24.5789) projected
  spline S1 degree 2 poles (42.4571, -24.5789) (42.1407, -24.5789) (41.6909, -24.658) (41.5376, -24.7816) knots 0 0 0 0.5 1 1 1 projected
  spline S2 degree 2 poles (41.5376, -24.7816) (41.3893, -24.9002) (41.246, -25.2166) (41.246, -25.4737) knots 0 0 0 0.5 1 1 1 projected
  spline S3 degree 2 poles (41.246, -25.4737) (41.246, -25.706) (41.4239, -26.0372) (41.6266, -26.1262) knots 0 0 0 0.5 1 1 1 projected
  spline S4 degree 2 poles (34.7752, -25.8493) (34.968, -26.1015) (35.4624, -26.319) (35.7293, -26.319) knots 0 0 0 0.5 1 1 1 projected
  spline S5 degree 2 poles (35.7293, -26.319) (36.0111, -26.319) (36.4708, -26.1163) (36.6833, -25.8592) knots 0 0 0 0.5 1 1 1 projected
  spline S6 degree 2 poles (36.6833, -25.8592) (36.8712, -25.622) (37.1035, -24.836) (37.1035, -24.2922) knots 0 0 0 0.5 1 1 1 projected
  spline S7 degree 2 poles (37.1035, -24.2922) (37.1035, -23.7287) (36.8811, -22.9872) (36.6883, -22.7351) knots 0 0 0 0.5 1 1 1 projected
  spline S8 degree 2 poles (36.6883, -22.7351) (36.4955, -22.483) (35.9962, -22.2655) (35.7293, -22.2655) knots 0 0 0 0.5 1 1 1 projected
  spline S9 degree 2 poles (35.7293, -22.2655) (35.4574, -22.2655) (34.9532, -22.4978) (34.7703, -22.745) knots 0 0 0 0.5 1 1 1 projected
  spline S10 degree 2 poles (34.7703, -22.745) (34.5726, -23.0119) (34.36, -23.7188) (34.36, -24.2922) knots 0 0 0 0.5 1 1 1 projected
  spline S11 degree 2 poles (34.36, -24.2922) (34.36, -24.8409) (34.5825, -25.6071) (34.7752, -25.8493) knots 0 0 0 0.5 1 1 1 projected
  spline S12 degree 2 poles (29.2684, -26.1509) (29.4167, -26.2201) (29.832, -26.23) (30.2423, -26.23) knots 0 0 0 0.5 1 1 1 projected
  line L3 (30.2423, -26.23) -> (30.3461, -26.23) projected
  line L4 (30.3461, -26.23) -> (30.3461, -24.9348) projected
  line L5 (30.3461, -24.9348) -> (30.1533, -24.9348) projected
  spline S13 degree 2 poles (30.1533, -24.9348) (29.7628, -24.9348) (29.4464, -24.9497) (29.2783, -25.0288) knots 0 0 0 0.5 1 1 1 projected
  spline S14 degree 2 poles (29.2783, -25.0288) (29.0954, -25.1177) (28.957, -25.4193) (28.957, -25.622) knots 0 0 0 0.5 1 1 1 projected
  spline S15 degree 2 poles (28.957, -25.622) (28.957, -25.7703) (29.1103, -26.0817) (29.2684, -26.1509) knots 0 0 0 0.5 1 1 1 projected
  spline S16 degree 2 poles (29.0312, -23.8275) (29.1696, -23.8819) (29.659, -23.8918) (30.0643, -23.8918) knots 0 0 0 0.5 1 1 1 projected
  line L6 (30.0643, -23.8918) -> (30.3461, -23.8918) projected
  line L7 (30.3461, -23.8918) -> (30.3461, -22.3545) projected
  line L8 (30.3461, -22.3545) -> (30.262, -22.3545) projected
  spline S17 degree 2 poles (30.262, -22.3545) (29.6688, -22.3545) (29.2141, -22.3693) (28.9768, -22.4731) knots 0 0 0 0.5 1 1 1 projected
  spline S18 degree 2 poles (28.9768, -22.4731) (28.7692, -22.567) (28.5764, -22.913) (28.5764, -23.1355) knots 0 0 0 0.5 1 1 1 projected
  spline S19 degree 2 poles (28.5764, -23.1355) (28.5764, -23.4222) (28.8038, -23.7435) (29.0312, -23.8275) knots 0 0 0 0.5 1 1 1 projected
  line L9 (7.2462, -25.6121) -> (7.8739, -23.5952) projected
  line L10 (7.8739, -23.5952) -> (6.6233, -23.5952) projected
  line L11 (6.6233, -23.5952) -> (7.2462, -25.6121) projected
  point P0 (25.0207, -3)
  constraints: 20 other
extrude "Extrusion57" cut sketch "Sketch48" against normal up to next
extrude "Extrusion58" cut sketch "Sketch40" against normal up to next contours A4 | A5
sketch "Sketch49" plane through (0, 0, 0) normal (0, -1, 0) x (1, 0, 0)
  line L0 (-22.6532, -3.8312) -> (-22.6532, -28.5716) projected
  line L1 (-22.6532, -28.5716) -> (-32.6532, -28.5716) projected
  line L2 (-20.1532, -3.7014) -> (-35.1532, -3.7014)
  line L3 (-35.1532, -3.7014) -> (-35.1532, -28.7014)
  line L4 (-35.1532, -28.7014) -> (-20.1532, -28.7014)
  line L5 (-20.1532, -28.7014) -> (-20.1532, -3.7014)
  line L6 (-20.1532, -3.7014) -> (-35.1532, -28.7014) construction
  line L7 (-35.1532, -3.7014) -> (-20.1532, -28.7014) construction
  point P0 (0, 0)
  point P1 (-27.6532, -16.2014)
  point P2 (-27.6532, -16.2014)
  dimension "d343" = 15
  dimension "d344" = 25
  constraints: 12 end point, 2 midpoint, 2 parallel, 1 horizontal, 1 perpendicular
  measures "d343" distance of L4.end L3.end
  measures "d344" distance of L3.end L2.end
extrude "Extrusion59" cut sketch "Sketch49" against normal up to next
body "Solid2"
